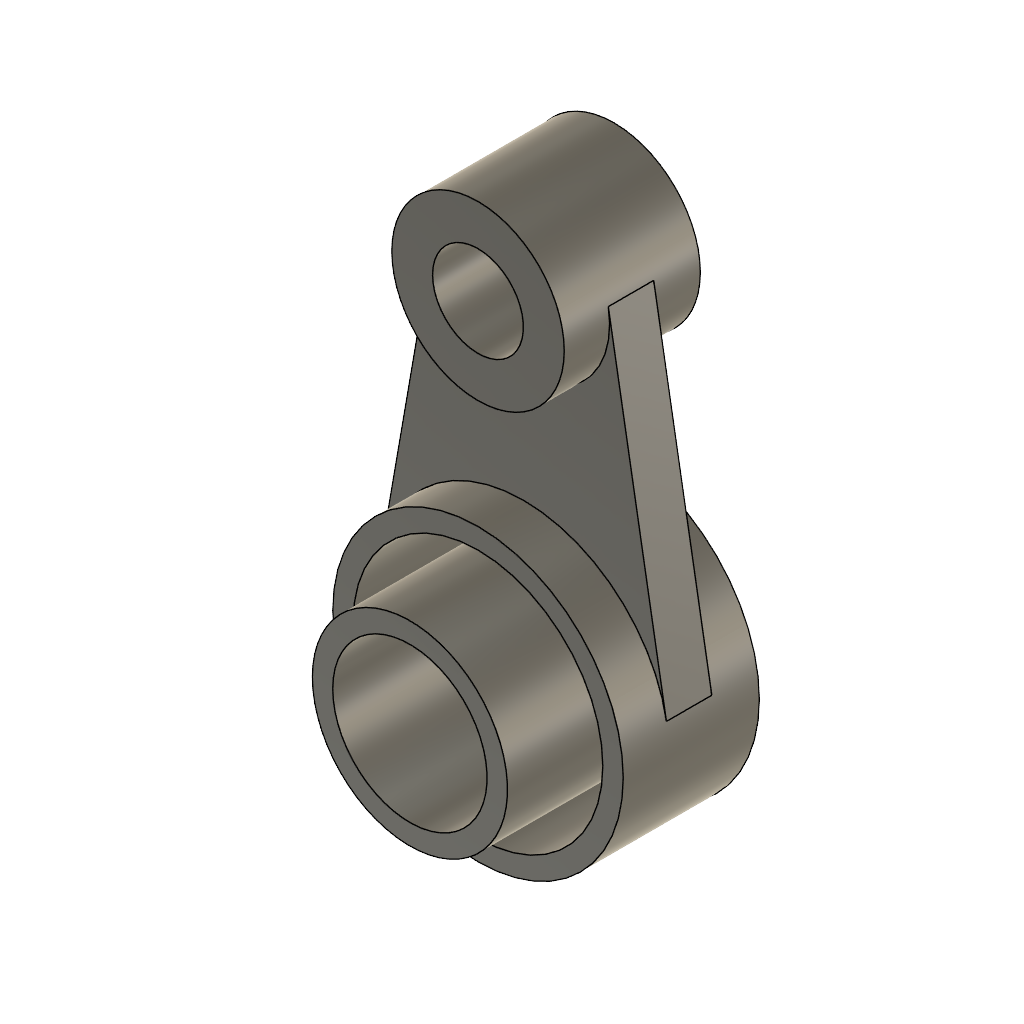
exercise 12 (Autodesk Fusion 360 design; units mm, degrees)
part number: 2026-10-07-17-04-14-943
Autodesk Fusion 360 part; units mm, degrees
sketch "Sketch1" plane through (0, 0, 0) normal (0, 1, 0) x (1, 0, 0)
  circle A0 centre (0, 0) radius 17
  circle A1 centre (0, 0) radius 21.5
  circle A2 centre (0, 0) radius 27.5
  circle A3 centre (0, 0) radius 32
  circle A4 centre (0, -75) radius 10
  circle A5 centre (0, -75) radius 19
  line L0 (-18.7124, -78.2933) -> (-31.5156, -5.5467)
  line L1 (18.7124, -78.2933) -> (31.5156, -5.5467)
  dimension "d1" = 34
  dimension "d2" = 43
  dimension "d3" = 55
  dimension "d4" = 64
  dimension "d5" = 20
  dimension "d6" = 38
  dimension "d7" = 75
  constraint coincident A0.centre A1.centre
  constraint concentric A2 A3
  constraint concentric A4 A5
  constraint coincident A5 L0.start
  constraint coincident A3 L0.end
  constraint coincident A5 L1.start
  constraint coincident A3 L1.end
  constraint tangent A5 L0
  constraint tangent A3 L0
  constraint tangent A5 L1
  constraint tangent A3 L1
  measures "d1" diameter of A0
  measures "d2" diameter of A1
  measures "d3" diameter of A2
  measures "d4" diameter of A3
  measures "d5" diameter of A4
  measures "d6" diameter of A5
  measures "d7" distance of A0.centre A4.centre
extrude "Extrude1" add sketch "Sketch1" along normal mid plane 30 contours A5 makes body 1
extrude "Extrude2" add sketch "Sketch1" against normal blind 30 separate body contours A1 makes body 2
extrude "Extrude3" add sketch "Sketch1" along normal mid plane 30 separate body contours A3 makes body 3
extrude "Extrude4" add sketch "Sketch1" along normal mid plane 10 contours A3 A5 L0 L1 bodies 1 3
